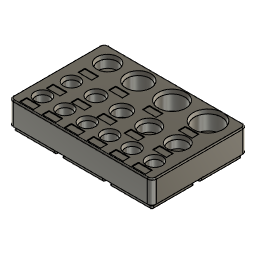
HarborFreightSocketHolder_Metric (Autodesk Fusion 360 design; units mm, degrees)
Autodesk Fusion 360 part; units mm, degrees
sketch "Sketch1" plane through (0, 0, 0) normal (0, 0, 1) x (1, 0, 0) in component "Blank Storage"
  line L0 (0, 42) -> (42, 42)
  line L1 (42, 42) -> (42, 0)
  line L2 (42, 0) -> (0, 0)
  line L3 (0, 0) -> (0, 42)
  line L4 (0, 42) -> (42, 0) construction
  line L5 (42, 21) -> (0, 21) construction
  line L6 (42, 14.5) -> (0, 14.5)
  line L7 (42, 27.5) -> (0, 27.5)
  line L8 (27.5, 42) -> (27.5, 0)
  line L9 (14.5, 42) -> (14.5, 0)
  line L10 (14.5, 14.5) -> (0, 0) construction
  circle A0 centre (8, 8) radius 1.5
  circle A1 centre (34, 8) radius 1.5
  circle A2 centre (34, 34) radius 1.5
  circle A3 centre (8, 34) radius 1.5
  circle A4 centre (8, 8) radius 3.25
  circle A5 centre (34, 8) radius 3.25
  circle A6 centre (34, 34) radius 3.25
  circle A7 centre (8, 34) radius 3.25
  point P0 (21, 21)
  dimension "d1" = 42
  dimension "d2" = 42
  dimension "d65" = 13
  dimension "d67" = 90
  dimension "d69" = 3
  dimension "d71" = 360
  dimension "d80" = 6.5
  dimension "d85" = 8
  constraint horizontal L0
  constraint perpendicular L0 L1
  constraint parallel L0 L2
  constraint parallel L1 L3
  constraint coincident L2.end L3.start
  constraint midpoint L1 L5.start
  constraint midpoint L3 L5.end
  constraint coincident L1 L6.start
  constraint coincident L3 L6.end
  constraint perpendicular L3 L6
  constraint symmetric L5 L6.start L7.start
  constraint symmetric L5 L6.end L7.end
  constraint midpoint L4 P0
  constraint coincident L9 L10.start
  constraint coincident L6 L10.start
  constraint concentric A0 A4
  constraint coincident L10 A0.centre
  measures "d1" distance of L1.end L2.end
  measures "d2" distance of L0.end L1.end
  measures "d65" distance of L6 L7
  measures "d69" diameter of A0
  measures "d80" diameter of A4
  measures "d85" distance of L2 A0.centre
extrude "Extrude1" add sketch "Sketch1" along normal blind 5 contours L0 L3 L7 L9 | L0 L7 L8 L9 | L3 L6 L7 L9 | L0 L1 L7 L8 | L6 L7 L8 L9 | L2 L3 L6 L9 | L1 L6 L7 L8 | L2 L6 L8 L9 | L1 L2 L6 L8 | A0 | A1 | A2 | A3 | A4 | A5 | A6 | A7 makes body 1 in component "Blank Storage"
ref_plane "WorkPlane1" through (21, 21, 2.5) normal (0, -1, 0) x (1, 0, 0) in component "Blank Storage"
sketch "Sketch2" plane through (0, 21, 0) normal (0, -1, 0) x (1, 0, 0) in component "Blank Storage"
  line L0 (42, 0) -> (0, 0)
  line L1 (0, 0) -> (0, 5)
  line L2 (3.2, 0) -> (2.4, 0.8)
  line L3 (3.2, 0) -> (0, 0) construction
  line L4 (2.4, 0.8) -> (2.4, 2.6)
  line L5 (2.4, 2.6) -> (0, 5)
  line L6 (0, 5) -> (-5.1222, 5)
  line L7 (-5.1222, 5) -> (-5.1222, -0.0937)
  line L8 (-5.1222, -0.0937) -> (0, 0)
  dimension "d39" = 45
  dimension "d40" = 45
  dimension "d41" = 0.8
  dimension "d43" = 5
  dimension "d112" = 2.4
  constraint horizontal L3
  constraint coincident L0 L2.start
  constraint perpendicular L0 L4
  constraint coincident L1 L5.end
  constraint coincident L0.end L1.start
  constraint coincident L1.end L5.end
  constraint perpendicular L1 L6
  constraint perpendicular L6 L7
  measures "d39" angle of L2 L3
  measures "d40" angle of L4 L5
  measures "d41" distance of L2.end L3
  measures "d43" distance of L3 L1.end
  measures "d112" horizontal distance of L0.end L2.end
sketch "Sketch3" plane through (0, 0, 0) normal (0, 0, -1) x (1, 0, 0)
  line L0 (42, 0) -> (0, 0)
  line L1 (0, 0) -> (0, -42)
  line L2 (0, -42) -> (42, -42)
  line L3 (42, -42) -> (42, 0)
  arc A0 (4, 0) -> (0, -4) centre (4, -4) ccw
  line L4 (0, -42) -> (42, 0) construction
  arc A1 (0, -38) -> (4, -42) centre (4, -38) ccw
  arc A2 (38, -42) -> (42, -38) centre (38, -38) ccw
  arc A3 (42, -4) -> (38, 0) centre (38, -4) ccw
  line L5 (0, -4) -> (0, -38)
  line L6 (4, -42) -> (38, -42)
  line L7 (42, -38) -> (42, -4)
  line L8 (38, 0) -> (4, 0)
  point P0 (21, -21)
  dimension "d37" = 360
  constraint coincident L1.end L2.start
  constraint coincident L0.start L3.end
  constraint midpoint L4 P0
sweep "Sweep1" cut profiles "Sketch2" path "Sketch3" along L8 A0 L5 A1 L6 A2 L7 A3 section 1 bodies 1 in component "Blank Storage"
extrude "Extrude3" [suppressed] in component "Blank Storage"
draft "Draft1" [suppressed] in component "Blank Storage"
extrude "Extrude4" cut sketch "Sketch1" along normal up to surface (5 mm away) contours A0 | A1 | A2 | A3 bodies 1 in component "Blank Storage"
extrude "Extrude5" cut sketch "Sketch1" along normal blind 2.4 contours A4 | A5 | A6 | A7 bodies 1 in component "Blank Storage"
chamfer "Chamfer1" distance 1.75 angle 45 4 edges at (33.4576, 6.6015, 2.4) (35.3985, 33.4576, 2.4) (8.5424, 35.3985, 2.4) (6.6015, 8.5424, 2.4) on bodies 1 in component "Blank Storage"
pattern_linear "R-Pattern1" count 3 spacing 42 along (1, 0, 0) count 2 spacing 42 along (0, 1, 0) of bodies 1 makes body 2 at (66.9668, 17.0068, 5) makes body 3 at (24.9668, 59.0068, 5) makes body 4 at (66.9668, 59.0068, 5) makes body 5 at (108.9668, 17.0068, 5) makes body 6 at (108.9668, 59.0068, 5) in component "Blank Storage"
sketch "Sketch4" plane through (0, 0, 5) normal (0, 0, 1) x (-1, 0, 0) in component "Blank Storage"
  line L0 (-4, 0) -> (-122, 0)
  line L1 (-126, -4) -> (-126, -80)
  line L2 (-122, -84) -> (-4, -84)
  line L3 (0, -80) -> (0, -4)
  arc A0 (0, -4) -> (-4, 0) centre (-4, -4) ccw
  arc A1 (-122, 0) -> (-126, -4) centre (-122, -4) ccw
  arc A2 (-126, -80) -> (-122, -84) centre (-122, -80) ccw
  arc A3 (-4, -84) -> (0, -80) centre (-4, -80) ccw
  line L4 (-122, -83.75) -> (-4, -83.75)
  arc A4 (-4, -83.75) -> (-0.25, -80) centre (-4, -80) ccw
  line L5 (-0.25, -80) -> (-0.25, -4)
  arc A5 (-0.25, -4) -> (-4, -0.25) centre (-4, -4) ccw
  line L6 (-4, -0.25) -> (-122, -0.25)
  arc A6 (-122, -0.25) -> (-125.75, -4) centre (-122, -4) ccw
  line L7 (-125.75, -4) -> (-125.75, -80)
  arc A7 (-125.75, -80) -> (-122, -83.75) centre (-122, -80) ccw
  point P0 (-126, 0)
  point P1 (0, -84)
  dimension "d44" = 126
  dimension "d45" = 84
  dimension "d48" = 4
  dimension "d49" = 4
  dimension "d50" = 4
  dimension "d51" = 4
  dimension "d118" = -0.25
  constraint horizontal L0
  constraint vertical L1
  constraint horizontal L2
  constraint vertical L3
  constraint coincident origin L0
  constraint coincident origin L3
  constraint tangent L0 A0
  constraint tangent L3 A0
  constraint coincident P0 L0
  constraint coincident P0 L1
  constraint tangent L0 A1
  constraint tangent L1 A1
  constraint tangent L1 A2
  constraint tangent L2 A2
  constraint coincident P1 L2
  constraint coincident P1 L3
  constraint tangent L2 A3
  constraint tangent L3 A3
  measures "d44" distance of origin P0
  measures "d45" distance of origin P1
  measures "d48" radius of A0
  measures "d49" radius of A1
  measures "d50" radius of A2
  measures "d51" radius of A3
extrude "Extrude2" add sketch "Sketch4" along normal blind 20 contours L0 L1 L2 L3 A0 A1 A2 A3 | L4 A4 L5 A5 L6 A6 L7 A7 bodies 1 5 6 3 4 2 in component "Blank Storage"
sketch "Sketch6" plane through (0, 0, 25) normal (0, 0, 1) x (-1, 0, 0)
  arc A0 (-4, -84) -> (0, -80) centre (-4, -80) ccw
  line L0 (0, -80) -> (0, -4)
  arc A1 (0, -4) -> (-4, 0) centre (-4, -4) ccw
  line L1 (-4, 0) -> (-122, 0)
  arc A2 (-122, 0) -> (-126, -4) centre (-122, -4) ccw
  line L2 (-126, -4) -> (-126, -80)
  arc A3 (-126, -80) -> (-122, -84) centre (-122, -80) ccw
  line L3 (-122, -84) -> (-4, -84)
  circle A4 centre (-13.7143, -16) radius 6
  circle A5 centre (-33.4286, -16) radius 6
  circle A6 centre (-53.1429, -16) radius 6
  circle A7 centre (-72.8571, -16) radius 6
  circle A8 centre (-92.5714, -16) radius 6
  circle A9 centre (-112.2857, -16) radius 6
  line L4 (0, -16) -> (-126, -16) construction
  line L5 (-126, -40) -> (0, -40) construction
  line L6 (0, -70) -> (-126, -70) construction
  circle A10 centre (-15.1667, -40) radius 6
  circle A11 centre (-36.8333, -40) radius 6.5
  circle A12 centre (-59.5, -40) radius 7
  circle A13 centre (-83.6667, -40) radius 8
  circle A14 centre (-108.8333, -40) radius 8
  circle A15 centre (-17.06, -70) radius 8.5
  circle A16 centre (-44.12, -70) radius 10
  circle A17 centre (-73.78, -70) radius 11.1
  circle A18 centre (-105.44, -70) radius 12
  line L7 (-11.06, -56) -> (-23.06, -56)
  line L8 (-23.06, -56) -> (-23.06, -50)
  line L9 (-23.06, -50) -> (-11.06, -50)
  line L10 (-11.06, -50) -> (-11.06, -56)
  line L11 (-11.06, -56) -> (-23.06, -50) construction
  line L12 (-23.06, -56) -> (-11.06, -50) construction
  line L13 (-38.12, -56) -> (-50.12, -56)
  line L14 (-50.12, -56) -> (-50.12, -50)
  line L15 (-50.12, -50) -> (-38.12, -50)
  line L16 (-38.12, -50) -> (-38.12, -56)
  line L17 (-38.12, -56) -> (-50.12, -50) construction
  line L18 (-50.12, -56) -> (-38.12, -50) construction
  line L19 (-67.78, -56) -> (-79.78, -56)
  line L20 (-79.78, -56) -> (-79.78, -50)
  line L21 (-79.78, -50) -> (-67.78, -50)
  line L22 (-67.78, -50) -> (-67.78, -56)
  line L23 (-67.78, -56) -> (-79.78, -50) construction
  line L24 (-79.78, -56) -> (-67.78, -50) construction
  line L25 (-99.44, -56) -> (-111.44, -56)
  line L26 (-111.44, -56) -> (-111.44, -50)
  line L27 (-111.44, -50) -> (-99.44, -50)
  line L28 (-99.44, -50) -> (-99.44, -56)
  line L29 (-99.44, -56) -> (-111.44, -50) construction
  line L30 (-111.44, -56) -> (-99.44, -50) construction
  line L31 (-105.44, -70) -> (-105.44, -53) construction
  line L32 (-105.44, -53) -> (-17.06, -53) construction
  line L33 (-17.06, -53) -> (-17.06, -70) construction
  line L34 (-44.12, -53) -> (-44.12, -70) construction
  line L35 (-73.78, -53) -> (-73.78, -70) construction
  line L36 (-102.8333, -30) -> (-114.8333, -30)
  line L37 (-114.8333, -30) -> (-114.8333, -24)
  line L38 (-114.8333, -24) -> (-102.8333, -24)
  line L39 (-102.8333, -24) -> (-102.8333, -30)
  line L40 (-102.8333, -30) -> (-114.8333, -24) construction
  line L41 (-114.8333, -30) -> (-102.8333, -24) construction
  line L42 (-77.6667, -30) -> (-89.6667, -30)
  line L43 (-89.6667, -30) -> (-89.6667, -24)
  line L44 (-89.6667, -24) -> (-77.6667, -24)
  line L45 (-77.6667, -24) -> (-77.6667, -30)
  line L46 (-77.6667, -30) -> (-89.6667, -24) construction
  line L47 (-89.6667, -30) -> (-77.6667, -24) construction
  line L48 (-65.5, -30) -> (-53.5, -30)
  line L49 (-53.5, -30) -> (-53.5, -24)
  line L50 (-53.5, -24) -> (-65.5, -24)
  line L51 (-65.5, -24) -> (-65.5, -30)
  line L52 (-65.5, -30) -> (-53.5, -24) construction
  line L53 (-53.5, -30) -> (-65.5, -24) construction
  line L54 (-42.8333, -24) -> (-30.8333, -24)
  line L55 (-30.8333, -24) -> (-30.8333, -30)
  line L56 (-30.8333, -30) -> (-42.8333, -30)
  line L57 (-42.8333, -30) -> (-42.8333, -24)
  line L58 (-42.8333, -24) -> (-30.8333, -30) construction
  line L59 (-30.8333, -24) -> (-42.8333, -30) construction
  line L60 (-21.1667, -24) -> (-9.1667, -24)
  line L61 (-9.1667, -24) -> (-9.1667, -30)
  line L62 (-9.1667, -30) -> (-21.1667, -30)
  line L63 (-21.1667, -30) -> (-21.1667, -24)
  line L64 (-21.1667, -24) -> (-9.1667, -30) construction
  line L65 (-9.1667, -24) -> (-21.1667, -30) construction
  line L66 (-118.2857, -8) -> (-106.2857, -8)
  line L67 (-106.2857, -8) -> (-106.2857, -2)
  line L68 (-106.2857, -2) -> (-118.2857, -2)
  line L69 (-118.2857, -2) -> (-118.2857, -8)
  line L70 (-118.2857, -8) -> (-106.2857, -2) construction
  line L71 (-106.2857, -8) -> (-118.2857, -2) construction
  line L72 (-98.5714, -8) -> (-86.5714, -8)
  line L73 (-86.5714, -8) -> (-86.5714, -2)
  line L74 (-86.5714, -2) -> (-98.5714, -2)
  line L75 (-98.5714, -2) -> (-98.5714, -8)
  line L76 (-98.5714, -8) -> (-86.5714, -2) construction
  line L77 (-86.5714, -8) -> (-98.5714, -2) construction
  line L78 (-78.8571, -2) -> (-66.8571, -2)
  line L79 (-66.8571, -2) -> (-66.8571, -8)
  line L80 (-66.8571, -8) -> (-78.8571, -8)
  line L81 (-78.8571, -8) -> (-78.8571, -2)
  line L82 (-78.8571, -2) -> (-66.8571, -8) construction
  line L83 (-66.8571, -2) -> (-78.8571, -8) construction
  line L84 (-59.1429, -8) -> (-47.1429, -8)
  line L85 (-47.1429, -8) -> (-47.1429, -2)
  line L86 (-47.1429, -2) -> (-59.1429, -2)
  line L87 (-59.1429, -2) -> (-59.1429, -8)
  line L88 (-59.1429, -8) -> (-47.1429, -2) construction
  line L89 (-47.1429, -8) -> (-59.1429, -2) construction
  line L90 (-39.4286, -8) -> (-27.4286, -8)
  line L91 (-27.4286, -8) -> (-27.4286, -2)
  line L92 (-27.4286, -2) -> (-39.4286, -2)
  line L93 (-39.4286, -2) -> (-39.4286, -8)
  line L94 (-39.4286, -8) -> (-27.4286, -2) construction
  line L95 (-27.4286, -8) -> (-39.4286, -2) construction
  line L96 (-7.7143, -8) -> (-19.7143, -8)
  line L97 (-19.7143, -8) -> (-19.7143, -2)
  line L98 (-19.7143, -2) -> (-7.7143, -2)
  line L99 (-7.7143, -2) -> (-7.7143, -8)
  line L100 (-7.7143, -8) -> (-19.7143, -2) construction
  line L101 (-19.7143, -8) -> (-7.7143, -2) construction
  line L102 (-108.8333, -27) -> (-15.1667, -27) construction
  line L103 (-112.2857, -5) -> (-13.7143, -5) construction
  line L104 (-108.8333, -27) -> (-108.8333, -40) construction
  line L105 (-83.6667, -27) -> (-83.6667, -40) construction
  line L106 (-59.5, -27) -> (-59.5, -40) construction
  line L107 (-36.8333, -27) -> (-36.8333, -40) construction
  line L108 (-15.1667, -27) -> (-15.1667, -40) construction
  line L109 (-13.7143, -5) -> (-13.7143, -16) construction
  line L110 (-33.4286, -5) -> (-33.4286, -16) construction
  line L111 (-53.1429, -5) -> (-53.1429, -16) construction
  line L112 (-72.8571, -5) -> (-72.8571, -16) construction
  line L113 (-92.5714, -5) -> (-92.5714, -16) construction
  line L114 (-112.2857, -5) -> (-112.2857, -16) construction
  point P0 (-8.56, -70)
  point P1 (-117.44, -70)
  point P2 (-116.8333, -40)
  point P3 (-9.1667, -40)
  point P4 (-25.56, -70)
  point P5 (-34.12, -70)
  point P6 (-54.12, -70)
  point P7 (-62.68, -70)
  point P8 (-84.88, -70)
  point P9 (-93.44, -70)
  point P10 (-21.1667, -40)
  point P11 (-30.3333, -40)
  point P12 (-43.3333, -40)
  point P13 (-52.5, -40)
  point P14 (-66.5, -40)
  point P15 (-75.6667, -40)
  point P16 (-91.6667, -40)
  point P17 (-100.8333, -40)
  point P18 (-17.06, -53)
  point P19 (-44.12, -53)
  point P20 (-73.78, -53)
  point P21 (-105.44, -53)
  point P22 (-108.8333, -27)
  point P23 (-83.6667, -27)
  point P24 (-59.5, -27)
  point P25 (-36.8333, -27)
  point P26 (-15.1667, -27)
  point P27 (-112.2857, -5)
  point P28 (-92.5714, -5)
  point P29 (-72.8571, -5)
  point P30 (-53.1429, -5)
  point P31 (-33.4286, -5)
  point P32 (-13.7143, -5)
  dimension "d123" = 12
  dimension "d124" = 12
  dimension "d125" = 12
  dimension "d126" = 12
  dimension "d127" = 12
  dimension "d128" = 12
  dimension "d130" = 13
  dimension "d131" = 14
  dimension "d132" = 16
  dimension "d133" = 16
  dimension "d134" = 17
  dimension "d135" = 20
  dimension "d136" = 22.2
  dimension "d137" = 24
  dimension "d138" = 126
  dimension "d140" = 19.7143
  dimension "d141" = 19.7143
  dimension "d142" = 19.7143
  dimension "d143" = 19.7143
  dimension "d144" = 19.7143
  dimension "d145" = 13.7143
  dimension "d157" = 12
  dimension "d160" = 8.56
  dimension "d161" = 8.56
  dimension "d162" = 8.56
  dimension "d163" = 8.56
  dimension "d165" = 9.1667
  dimension "d166" = 9.1667
  dimension "d167" = 9.1667
  dimension "d168" = 9.1667
  dimension "d169" = 9.1667
  dimension "d173" = 30
  dimension "d174" = 24
  dimension "d176" = 16
  dimension "d181" = 6
  dimension "d183" = 12
  dimension "d184" = 17
  dimension "d185" = 13
  dimension "d186" = 11
  constraint coincident L0 L4.start
  constraint coincident L2 L4.end
  constraint perpendicular L2 L4
  constraint coincident L2 L5.start
  constraint coincident L0 L5.end
  constraint perpendicular L0 L5
  constraint coincident L0 L6.start
  constraint coincident L2 L6.end
  constraint perpendicular L2 L6
  constraint coincident L5 A10.centre
  constraint coincident L5 A11.centre
  constraint coincident L5 A12.centre
  constraint coincident L5 A13.centre
  constraint coincident L5 A14.centre
  constraint coincident L6 A15.centre
  constraint coincident L6 A16.centre
  constraint coincident L6 A17.centre
  constraint coincident L6 A18.centre
  constraint coincident A4.centre L4
  constraint coincident A5.centre L4
  constraint coincident A6.centre L4
  constraint coincident A7.centre L4
  constraint coincident A8.centre L4
  constraint coincident A9.centre L4
  constraint coincident A15 P0
  constraint coincident L6 P0
  constraint coincident A18 P1
  constraint coincident L6 P1
  constraint coincident A14 P2
  constraint coincident L5 P2
  constraint coincident L5 P3
  constraint coincident A10 P3
  constraint coincident L6 P4
  constraint coincident A15 P4
  constraint coincident L6 P5
  constraint coincident A16 P5
  constraint coincident A16 P6
  constraint coincident L6 P6
  constraint coincident A17 P7
  constraint coincident L6 P7
  constraint coincident A17 P8
  constraint coincident L6 P8
  constraint coincident A18 P9
  constraint coincident L6 P9
  constraint coincident A10 P10
  constraint coincident L5 P10
  constraint coincident A11 P11
  constraint coincident L5 P11
  constraint coincident A11 P12
  constraint coincident L5 P12
  constraint coincident A12 P13
  constraint coincident L5 P13
  constraint coincident A12 P14
  constraint coincident L5 P14
  constraint coincident A13 P15
  constraint coincident L5 P15
  constraint coincident A13 P16
  constraint coincident L5 P16
  constraint coincident A14 P17
  constraint coincident L5 P17
  constraint horizontal L7
  constraint perpendicular L7 L8
  constraint parallel L7 L9
  constraint parallel L8 L10
  constraint coincident L11 P18
  constraint coincident L12 P18
  constraint horizontal L13
  constraint perpendicular L13 L14
  constraint parallel L13 L15
  constraint parallel L14 L16
  constraint coincident L17 P19
  constraint coincident L18 P19
  constraint horizontal L19
  constraint perpendicular L19 L20
  constraint parallel L19 L21
  constraint parallel L20 L22
  constraint coincident L23 P20
  constraint coincident L24 P20
  constraint horizontal L25
  constraint perpendicular L25 L26
  constraint parallel L25 L27
  constraint parallel L26 L28
  constraint coincident L29 P21
  constraint coincident L30 P21
  constraint coincident A18.centre L31.start
  constraint coincident P21 L31.end
  constraint coincident P18 L32.end
  constraint vertical L31
  constraint horizontal L32
  constraint equal L20 L26
  constraint equal L14 L26
  constraint equal L8 L26
  constraint equal L19 L25
  constraint equal L13 L25
  constraint equal L7 L25
  constraint coincident A15.centre L33.end
  constraint coincident P19 L34.start
  constraint coincident A16.centre L34.end
  constraint coincident P20 L35.start
  constraint coincident A17.centre L35.end
  constraint vertical L35
  constraint vertical L34
  constraint vertical L33
  constraint coincident P19 L32
  constraint coincident P20 L32
  constraint horizontal L36
  constraint perpendicular L36 L37
  constraint parallel L36 L38
  constraint parallel L37 L39
  constraint coincident L40 P22
  constraint coincident L41 P22
  constraint horizontal L42
  constraint perpendicular L42 L43
  constraint parallel L42 L44
  constraint parallel L43 L45
  constraint coincident L46 P23
  constraint coincident L47 P23
  constraint horizontal L48
  constraint perpendicular L48 L49
  constraint parallel L48 L50
  constraint parallel L49 L51
  constraint coincident L52 P24
  constraint coincident L53 P24
  constraint horizontal L54
  constraint perpendicular L54 L55
  constraint parallel L54 L56
  constraint parallel L55 L57
  constraint coincident L58 P25
  constraint coincident L59 P25
  constraint horizontal L60
  constraint perpendicular L60 L61
  constraint parallel L60 L62
  constraint parallel L61 L63
  constraint coincident L64 P26
  constraint coincident L65 P26
  constraint horizontal L66
  constraint perpendicular L66 L67
  constraint parallel L66 L68
  constraint parallel L67 L69
  constraint coincident L70 P27
  constraint coincident L71 P27
  constraint horizontal L72
  constraint perpendicular L72 L73
  constraint parallel L72 L74
  constraint parallel L73 L75
  constraint coincident L76 P28
  constraint coincident L77 P28
  constraint horizontal L78
  constraint perpendicular L78 L79
  constraint parallel L78 L80
  constraint parallel L79 L81
  constraint coincident L82 P29
  constraint coincident L83 P29
  constraint horizontal L84
  constraint perpendicular L84 L85
  constraint parallel L84 L86
  constraint parallel L85 L87
  constraint coincident L88 P30
  constraint coincident L89 P30
  constraint horizontal L90
  constraint perpendicular L90 L91
  constraint parallel L90 L92
  constraint parallel L91 L93
  constraint coincident L94 P31
  constraint coincident L95 P31
  constraint horizontal L96
  constraint perpendicular L96 L97
  constraint parallel L96 L98
  constraint parallel L97 L99
  constraint coincident L100 P32
  constraint coincident L101 P32
  constraint equal L26 L37
  constraint equal L37 L43
  constraint equal L37 L51
  constraint equal L37 L57
  constraint equal L37 L63
  constraint equal L26 L69
  constraint equal L69 L75
  constraint equal L69 L81
  constraint equal L69 L87
  constraint equal L69 L93
  constraint equal L69 L97
  constraint equal L25 L36
  constraint equal L36 L42
  constraint equal L36 L48
  constraint equal L36 L56
  constraint equal L36 L62
  constraint equal L25 L66
  constraint equal L66 L72
  constraint equal L66 L80
  constraint equal L66 L84
  constraint equal L66 L90
  constraint equal L66 L96
  constraint coincident P22 L102.start
  constraint coincident P26 L102.end
  constraint coincident P27 L103.start
  constraint coincident P32 L103.end
  constraint perpendicular L91 L103
  constraint coincident P23 L102
  constraint coincident P24 L102
  constraint coincident P25 L102
  constraint coincident P28 L103
  constraint coincident P29 L103
  constraint coincident P30 L103
  constraint coincident P31 L103
  constraint horizontal L102
  constraint coincident A14.centre L104.end
  constraint coincident P23 L105.start
  constraint coincident A13.centre L105.end
  constraint coincident P24 L106.start
  constraint coincident A12.centre L106.end
  constraint coincident P25 L107.start
  constraint coincident A11.centre L107.end
  constraint coincident A10.centre L108.end
  constraint coincident A4.centre L109.end
  constraint coincident P31 L110.start
  constraint coincident A5.centre L110.end
  constraint coincident P30 L111.start
  constraint coincident A6.centre L111.end
  constraint coincident P29 L112.start
  constraint coincident A7.centre L112.end
  constraint coincident P28 L113.start
  constraint coincident A8.centre L113.end
  constraint coincident A9.centre L114.end
  constraint vertical L104
  constraint vertical L105
  constraint vertical L106
  constraint vertical L107
  constraint vertical L108
  constraint vertical L114
  constraint vertical L113
  constraint vertical L112
  constraint vertical L111
  constraint vertical L110
  constraint vertical L109
  measures "d123" diameter of A4
  measures "d124" diameter of A5
  measures "d125" diameter of A6
  measures "d126" diameter of A7
  measures "d127" diameter of A8
  measures "d128" diameter of A9
  measures "d130" diameter of A11
  measures "d131" diameter of A12
  measures "d132" diameter of A13
  measures "d133" diameter of A14
  measures "d134" diameter of A15
  measures "d135" diameter of A16
  measures "d136" diameter of A17
  measures "d137" diameter of A18
  measures "d138" distance of L4.start L4.end
  measures "d140" distance of A4.centre A5.centre
  measures "d141" distance of A5.centre A6.centre
  measures "d142" distance of A6.centre A7.centre
  measures "d143" distance of A7.centre A8.centre
  measures "d144" distance of A8.centre A9.centre
  measures "d145" distance of A4.centre L4.start
  measures "d157" diameter of A10
  measures "d160" distance of L6.start P0
  measures "d161" distance of P4 P5
  measures "d162" distance of P6 P7
  measures "d163" distance of P8 P9
  measures "d165" distance of L5.end P3
  measures "d166" distance of P10 P11
  measures "d167" distance of P12 P13
  measures "d168" distance of P14 P15
  measures "d169" distance of P16 P17
  measures "d173" distance of L5 L6
  measures "d174" distance of L4 L5
  measures "d176" distance of L1 L4
  measures "d181" distance of L25.end L26.end
  measures "d183" distance of L25.start L25.end
  measures "d184" distance of L6 L32
  measures "d185" distance of A14.centre P22
  measures "d186" distance of L4 P27
extrude "Extrude3'" cut sketch "Sketch6" against normal blind 10 contours A4 | A5 | A6 | A7 | A8 | A9 | A10 | A11 | A12 | A13 | A14 | A15 bodies 1 in component "Blank Storage"
extrude "Extrude4'" cut sketch "Sketch6" against normal blind 16 contours A16 | A17 | A18 bodies 1 in component "Blank Storage"
extrude "Extrude5'" cut sketch "Sketch6" against normal blind 0.6 contours L7 L8 L9 L10 | L13 L14 L15 L16 | L19 L20 L21 L22 | L25 L26 L27 L28 | L36 L37 L38 L39 | L42 L43 L44 L45 | L48 L49 L50 L51 | L54 L55 L56 L57 | L60 L61 L62 L63 | L66 L67 L68 L69 | L72 L73 L74 L75 | L78 L79 L80 L81 | L84 L85 L86 L87 | L90 L91 L92 L93 | L96 L97 L98 L99 bodies 1 in component "Blank Storage"
chamfer "Chamfer2" distance 1 distance2 3 15 edges at (116.6279, 65.6606, 25) (84.1288, 65.9861, 25) (53.4433, 66.3838, 25) (24.9848, 66.9263, 25) (20.7606, 37.8303, 25) (42.8935, 37.6495, 25) (66.0263, 37.4687, 25) (91.1253, 37.1071, 25) (116.292, 37.1071, 25) (117.8797, 13.8303, 25) (98.1654, 13.8303, 25) (78.4511, 13.8303, 25) (58.7368, 13.8303, 25) (39.0225, 13.8303, 25) (19.3082, 13.8303, 25) measured on face at (122.9444, 41.3333, 25) measured on face at (122.9444, 41.3333, 25) measured on face at (122.9444, 41.3333, 25) measured on face at (122.9444, 41.3333, 25) measured on face at (122.9444, 41.3333, 25) measured on face at (122.9444, 41.3333, 25) measured on face at (122.9444, 41.3333, 25) measured on face at (122.9444, 41.3333, 25) measured on face at (122.9444, 41.3333, 25) measured on face at (122.9444, 41.3333, 25) measured on face at (122.9444, 41.3333, 25) measured on face at (122.9444, 41.3333, 25) measured on face at (122.9444, 41.3333, 25) measured on face at (122.9444, 41.3333, 25) measured on face at (122.9444, 41.3333, 25) on bodies 1 in component "Blank Storage"
fillet "Fillet2" radius 1 8 edges at (0, 42, 25) (1.1716, 1.1716, 25) (63, 0, 25) (124.8284, 1.1716, 25) (126, 42, 25) (124.8284, 82.8284, 25) (63, 84, 25) (1.1716, 82.8284, 25) on bodies 1 in component "Blank Storage"
component "Blank Storage" placed x (1, 0, 0) y (0, 1, 0) z (0, 0, 1) at (0, 0, 0)
equation "d1 = slotDimension"
equation "d2 = slotDimension"
equation "d3 = nestingDepth"
equation "slotsWide = 3"
equation "slotsHigh = 1 / 2"
equation "slotsDeep = 2"
equation "slotDimension = 42 mm"
equation "nestingDepth = 5 mm"
equation "nestingRimWidth = 2.4 mm"
equation "nestingClearance = 0.25 mm"
equation "cornerFillet = 4 mm"
equation "d31 = slotsWide"
equation "d32 = slotsDeep"
equation "d33 = slotDimension"
equation "d34 = slotDimension"
equation "d38 = -slotDimension / 2"
equation "d43 = nestingDepth"
equation "d44 = slotDimension * slotsWide"
equation "d45 = slotDimension * slotsDeep"
equation "d48 = cornerFillet"
equation "d49 = cornerFillet"
equation "d50 = cornerFillet"
equation "d51 = cornerFillet"
equation "ledStripWidth = 13 mm"
equation "ledSlotHeight = 4 mm"
equation "d65 = ledStripWidth"
equation "screwTightDiameter = 3 mm"
equation "d69 = screwTightDiameter"
equation "d72 = ledSlotHeight"
equation "magnetDiameter = 6.5 mm"
equation "magnetThiccness = 2.4 mm"
equation "d80 = magnetDiameter"
equation "d81 = magnetThiccness"
equation "wallThiccness = 1.2 mm"
equation "d112 = nestingRimWidth"
equation "d124 = d123"
equation "d125 = d123"
equation "d126 = d123"
equation "d127 = d123"
equation "d128 = d123"
equation "d139 = d138 / 6"
equation "d140 = d145 + d124 / 2"
equation "d141 = d140"
equation "d142 = d140"
equation "d143 = d140"
equation "d144 = d140"
equation "d145 = ( d138 - d123 * 6 ) / 7 + d123 / 2"
equation "d146 = d138 / 5"
equation "d151 = d138 / 4"
equation "d152 = d151"
equation "d157 = d123"
equation "d160 = ( ( d138 - d134 - d135 - d136 - d137 ) / 5 mm ) * 1 mm"
equation "d161 = d160"
equation "d162 = d160"
equation "d163 = d160"
equation "d165 = ( d138 - d157 - d130 - d131 - d132 - d133 ) / 6"
equation "d166 = d165"
equation "d167 = d166"
equation "d168 = d167"
equation "d169 = d168"
equation "d173 = ( d137 / 2 + d133 / 2 ) + LabelHeight"
equation "d174 = ( d133 / 2 + d128 / 2 ) + LabelHeight"
equation "LabelHeight = 10 mm"
equation "d176 = d128 / 2 + LabelHeight"
equation "d184 = ( d173 - d137 / 2 - d133 / 2 - d181 ) / 2 + d137 / 2 + d181 / 2"
equation "d185 = ( d174 - d133 / 2 - d181 - d128 / 2 ) / 2 + d133 / 2 + d181 / 2"
equation "d186 = ( d176 - d128 / 2 - d181 ) / 2 + d128 / 2 + d181 / 2"
named bodies: "Body1 (1)"
